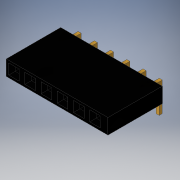
# Autodesk Inventor part: Right-Angle Female Header
Saved by Autodesk Inventor 2016 (Build 200138000, 138)
## iProperties
Created: 2015-11-30
Part Number: Right-Angle Female Header
Material: Generic
Document SubType Name: Modeling
Designer: Spooner
Density: 1 g/cm^3
Appearance: Black
Author: Spooner
Autodesk Inventor part; units mm, degrees
ref_plane "YZ Plane" through (0, 0, 0) normal (1, 0, 0) x (0, 1, 0)
ref_plane "XZ Plane" through (0, 0, 0) normal (0, 1, 0) x (-1, 0, 0)
ref_plane "XY Plane" through (0, 0, 0) normal (0, 0, 1) x (1, 0, 0)
sketch "Sketch1" plane through (0, 0, 0) normal (0, 0, 1) x (1, 0, 0)
  line L0 (0, 0) -> (15.9258, 0)
  line L1 (15.9258, 0) -> (15.9258, 2.3876)
  line L2 (15.9258, 2.3876) -> (0, 2.3876)
  line L3 (0, 2.3876) -> (0, 0)
  dimension "d0" = 15.9258
  dimension "d1" = 2.3876
  constraints: 8 end point, 2 parallel, 1 horizontal, 1 perpendicular
  measures "d0" distance of L1.end L2.end
  measures "d1" distance of L2.end L0.start
extrude "Extrusion1" add sketch "Sketch1" against normal blind 8.5217
sketch "Sketch2" plane through (0, 0, 0) normal (0, 0, 1) x (1, 0, 0)
  line L0 (0.8763, 1.5113) -> (1.5113, 1.5113)
  line L1 (1.5113, 1.5113) -> (1.5113, 0.8763)
  line L2 (1.5113, 0.8763) -> (0.8763, 0.8763)
  line L3 (0.8763, 0.8763) -> (0.8763, 1.5113)
  line L4 (0, 2.3876) -> (0, 0) projected
  line L5 (15.9258, 2.3876) -> (0, 2.3876) projected
  point P0 (0, 1.1938)
  point P1 (0.8763, 1.1938)
  dimension "d4" = 0.635
  dimension "d5" = 0.8763
  dimension "d6" = 0.8763
  constraints: 8 end point, 2 midpoint, 2 parallel, 2 perpendicular, 1 horizontal, 1 horizontal alignment
  measures "d4" distance of L0.end L0.start
  measures "d5" distance between parallel lines of L0 L5
  measures "d6" distance from line of point (0.876, 1.194) L4
extrude "Extrusion2" cut sketch "Sketch2" against normal blind 7.62
chamfer "Chamfer1" distance 0.508 angle 45 4 edges at (1.1938, 1.5113, 0) (0.8763, 1.1938, 0) (1.1938, 0.8763, 0) (1.5113, 1.1938, 0)
ref_plane "Work Plane1" through (1.1938, 0.8763, -7.62) normal (1, 0, 0) x (0, 0, -1)
sketch "Sketch3" plane through (1.1938, 0.8763, -7.62) normal (1, 0, 0) x (0, 0, -1)
  line L0 (0.9017, 1.5113) -> (0.9017, -0.8763) projected
  line L1 (0.9017, 0.5588) -> (2.6797, 0.5588)
  line L2 (2.6797, 0.5588) -> (2.6797, -4.1275)
  line L3 (2.6797, -4.1275) -> (2.1971, -4.1275)
  line L4 (2.1971, -4.1275) -> (2.1971, 0.0762)
  line L5 (2.1971, 0.0762) -> (0.9017, 0.0762)
  line L6 (-7.62, -0.8763) -> (0.9017, -0.8763) projected
  dimension "d15" = 0.4826
  dimension "d16" = 0.4826
  dimension "d17" = 0.9525
  dimension "d18" = 0.9525
  dimension "d19" = 1.778
  dimension "d20" = 3.2512
  constraints: 10 end point, 4 perpendicular, 2 point on line, 1 horizontal
  measures "d15" distance between parallel lines of L4 L2
  measures "d16" distance between parallel lines of L5 L1
  measures "d17" distance from line of L1 L0.start
  measures "d18" distance from line of L0.end L5
  measures "d19" distance of L1.start L1.end
  measures "d20" distance between parallel lines of L6 L3
extrude "Extrusion3" add sketch "Sketch3" along normal mid plane 0.4826
chamfer "Chamfer2" distance 0.127 angle 45 4 edges at (0.9525, -3.2512, -10.0584) (1.1938, -3.2512, -9.8171) (1.1938, -3.2512, -10.2997) (1.4351, -3.2512, -10.0584)
pattern_linear "Rectangular Pattern1" count 6 spacing 2.54 along (1, 0, 0) of "Extrusion2", "Chamfer1", "Extrusion3", "Chamfer2"
equation "\"d6\" = d5"
equation "\"d16\" = d15"
equation "\"d17\" = d18"
body "Solid1"
